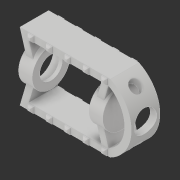
# Autodesk Inventor part: Pedal
Saved by Autodesk Inventor 2019 (Build 230136000, 136)
## iProperties
Created: 2020-06-01
Part Number: Pedal
Material: Generic
Document SubType Name: Modeling
Designer: 18186
Density: 1 g/cm^3
Appearance: Default
Author: 18186
Autodesk Inventor part; units mm, degrees
sketch "Sketch1" plane through (0, 0, 0) normal (0, 0, 1) x (1, 0, 0)
  line L0 (40, -30) -> (-40, -30)
  line L1 (-40, -30) -> (-40, 30) construction
  line L2 (-40, 30) -> (40, 30)
  line L3 (40, 30) -> (40, -30) construction
  line L4 (40, -30) -> (-40, 30) construction
  line L5 (-40, -30) -> (40, 30) construction
  line L6 (40, 30) -> (31.2306, 0)
  line L7 (31.2306, 0) -> (40, -30)
  line L8 (0, 0) -> (0, 5.5495) construction
  line L9 (-40, 30) -> (-31.2306, 0)
  line L10 (-31.2306, 0) -> (-40, -30)
  line L11 (-32.2696, 24.2022) -> (32.2696, 24.2022)
  line L12 (32.2696, 24.2022) -> (25.195, 0)
  line L13 (21.0953, 0) -> (28.6046, 0) construction
  line L14 (-32.2696, -24.2022) -> (32.2696, -24.2022)
  line L15 (32.2696, -24.2022) -> (25.195, 0)
  line L16 (-32.2696, 24.2022) -> (-25.195, 0)
  line L17 (-32.2696, -24.2022) -> (-25.195, 0)
  dimension "d0" = 80
  dimension "d1" = 60
  constraints: 36 end point, 4 symmetric about line, 3 horizontal, 3 parallel, 3 point on line, 2 midpoint, 1 perpendicular, 1 vertical
  measures "d0" distance of L1.end L2.end
  measures "d1" distance of L0.end L1.end
extrude "Extrusion1" add sketch "Sketch1" along normal blind 25.4
ref_plane "Work Plane2" through (-31.2306, 0, 0) normal (-1, 0, 0) x (0, 0, 1)
ref_plane "Work Plane1" through (-31.2306, 0, 0) normal (0, 1, 0) x (0, 0, 1)
sketch "Sketch2" plane through (-31.2306, 0, 0) normal (-1, 0, 0) x (0, 0, 1)
  line L0 (0, 0) -> (25.4, 0) projected
  circle A0 centre (12.7, 0) radius 16.7045
  dimension "d5" = 33.409
  constraints: 1 centre point, 1 midpoint
  measures "d5" diameter of A0
extrude "Extrusion2" add sketch "Sketch2" along normal mid plane 12.0904
sketch "Sketch3" plane through (-37.2758, 0, 12.7) normal (-1, 0, 0) x (0, 0, 1)
  point P0 (-12.7, 0)
sketch "Sketch4" plane through (-37.2758, 0, 12.7) normal (-1, 0, 0) x (0, 0, 1)
  circle A0 centre (0, 0) radius 14.1645
  dimension "d8" = 28.329
  constraints: 1 centre point
  measures "d8" diameter of A0
extrude "Extrusion3" cut sketch "Sketch4" against normal blind 9
sketch "Sketch5" plane through (-40, -30, 0) normal (0, -1, 0) x (1, 0, 0)
  line L0 (40, 25.4) -> (40, 0) construction
  constraints: 2 end point, 1 vertical
sketch "Sketch6" plane through (-40, 30, 0) normal (0, 1, 0) x (1, 0, 0)
  line L0 (40, -25.4) -> (40, 0) construction
  constraints: 2 end point, 1 vertical
ref_plane "Work Plane3" through (0, -30, 25.4) normal (1, 0, 0) x (0, 0, -1)
mirror "Mirror1" about plane through (0, -30, 25.4) normal (1, 0, 0) of "Extrusion2"
sketch "Sketch7" plane through (25.1854, 0, 12.7) normal (-1, 0, 0) x (0, 0, 1)
  circle A0 centre (0, 0) radius 14.1645
  point P0 (-12.7, 0)
  dimension "d11" = 28.329
  constraints: 1 centre point
  measures "d11" diameter of A0
extrude "Extrusion4" cut sketch "Sketch7" against normal blind 9
sketch "Sketch8" plane through (-28.2758, 0, 12.7) normal (-1, 0, 0) x (0, 0, 1)
  circle A0 centre (0, 0) radius 10
  point P0 (-12.7, 0)
  dimension "d14" = 20
  constraints: 1 centre point
  measures "d14" diameter of A0
extrude "Extrusion5" cut sketch "Sketch8" against normal blind 9
sketch "Sketch9" plane through (0, 0, 25.4) normal (0, 0, 1) x (1, 0, 0)
  arc A0 (40, -30) -> (40, 30) centre (25.1772, 0) ccw
  line L0 (32.2696, -24.2022) -> (38.3052, -24.2022) construction
  line L1 (32.2696, 24.2022) -> (38.3052, 24.2022) construction
  arc A1 (38.3052, -24.2022) -> (38.3052, 24.2022) centre (25.1772, 0) ccw
  line L2 (38.3052, -24.2022) -> (40, -30)
  line L3 (38.3052, 24.2022) -> (40, 30)
  point P0 (0, 0)
  constraints: 8 end point, 4 point on circle, 2 centre point, 2 horizontal, 1 concentric
extrude "Extrusion6" add sketch "Sketch9" against normal blind 25.4
ref_plane "Work Plane4" through (62.6758, 0, 12.7) normal (1, 0, 0) x (0, 0, -1)
sketch "Sketch10" plane through (62.6758, 0, 12.7) normal (1, 0, 0) x (0, 0, -1)
  circle A0 centre (0, 0) radius 10
  point P0 (12.7, 0)
  constraints: 1 centre point
extrude "Extrusion7" cut sketch "Sketch10" against normal blind 22.225
ref_plane "Work Plane5" through (40, 30, 0) normal (0.443, 0.8965, 0) x (-0.8965, 0.443, 0)
sketch "Sketch11" plane through (40, 30, 0) normal (0.443, 0.8965, 0) x (-0.8965, 0.443, 0)
  circle A0 centre (-11.6035, 12.5893) radius 5.1558
  point P0 (22.5723, 0)
  constraints: 1 centre point
extrude "Extrusion8" cut sketch "Sketch11" against normal blind 14.2875
ref_plane "Work Plane6" through (-40, 0, 25.4) normal (0, 1, 0) x (1, 0, 0)
mirror "Mirror2" about plane through (-40, 0, 25.4) normal (0, 1, 0) of "Extrusion8"
sketch "Sketch12" plane through (0, 0, 25.4) normal (0, 0, 1) x (1, 0, 0)
  line L0 (-32.2696, -24.2022) -> (-32.2696, -30) construction
  line L1 (-39.1526, -27.1011) -> (44.8049, -27.1011) construction
  line L2 (37.8474, -24.5611) -> (32.7674, -24.5611)
  line L3 (32.7674, -24.5611) -> (32.7674, -29.6411)
  line L4 (32.7674, -29.6411) -> (37.8474, -29.6411)
  line L5 (37.8474, -29.6411) -> (37.8474, -24.5611)
  line L6 (37.8474, -24.5611) -> (32.7674, -29.6411) construction
  line L7 (32.7674, -24.5611) -> (37.8474, -29.6411) construction
  line L8 (32.7674, -27.1011) -> (19.0514, -27.1011) construction
  line L9 (16.5114, -24.5611) -> (21.5914, -24.5611)
  line L10 (21.5914, -24.5611) -> (21.5914, -29.6411)
  line L11 (21.5914, -29.6411) -> (16.5114, -29.6411)
  line L12 (16.5114, -29.6411) -> (16.5114, -24.5611)
  line L13 (16.5114, -24.5611) -> (21.5914, -29.6411) construction
  line L14 (21.5914, -24.5611) -> (16.5114, -29.6411) construction
  line L15 (16.5114, -27.1011) -> (2.7954, -27.1011) construction
  line L16 (0.2554, -24.5611) -> (5.3354, -24.5611)
  line L17 (5.3354, -24.5611) -> (5.3354, -29.6411)
  line L18 (5.3354, -29.6411) -> (0.2554, -29.6411)
  line L19 (0.2554, -29.6411) -> (0.2554, -24.5611)
  line L20 (0.2554, -24.5611) -> (5.3354, -29.6411) construction
  line L21 (5.3354, -24.5611) -> (0.2554, -29.6411) construction
  line L22 (0.2554, -27.1011) -> (-13.4606, -27.1011) construction
  line L23 (-16.0006, -24.5611) -> (-10.9206, -24.5611)
  line L24 (-10.9206, -24.5611) -> (-10.9206, -29.6411)
  line L25 (-10.9206, -29.6411) -> (-16.0006, -29.6411)
  line L26 (-16.0006, -29.6411) -> (-16.0006, -24.5611)
  line L27 (-16.0006, -24.5611) -> (-10.9206, -29.6411) construction
  line L28 (-10.9206, -24.5611) -> (-16.0006, -29.6411) construction
  line L29 (-16.0006, -27.1011) -> (-29.7166, -27.1011) construction
  line L30 (-32.2566, -24.5611) -> (-27.1766, -24.5611)
  line L31 (-27.1766, -24.5611) -> (-27.1766, -29.6411)
  line L32 (-27.1766, -29.6411) -> (-32.2566, -29.6411)
  line L33 (-32.2566, -29.6411) -> (-32.2566, -24.5611)
  line L34 (-32.2566, -24.5611) -> (-27.1766, -29.6411) construction
  line L35 (-27.1766, -24.5611) -> (-32.2566, -29.6411) construction
  point P0 (0, 0)
  point P1 (35.3074, -27.1011)
  dimension "d24" = 5.08
  dimension "d25" = 5.08
  dimension "d26" = 13.716
  dimension "d27" = 5.08
  dimension "d28" = 5.08
  dimension "d29" = 13.716
  dimension "d30" = 5.08
  dimension "d31" = 5.08
  dimension "d32" = 13.716
  dimension "d33" = 5.08
  dimension "d34" = 5.08
  dimension "d35" = 13.716
  dimension "d36" = 5.08
  dimension "d37" = 5.08
  constraints: 72 end point, 14 midpoint, 10 parallel, 7 horizontal, 5 perpendicular, 5 point on line, 2 vertical
  measures "d24" distance of L4.end L3.end
  measures "d25" distance of L3.end L2.end
  measures "d26" distance of L8.start L8.end
  measures "d27" distance of L10.end L11.end
  measures "d28" distance of L9.end L10.end
  measures "d29" distance of L15.start L15.end
  measures "d30" distance of L17.end L18.end
  measures "d31" distance of L16.end L17.end
  measures "d32" distance of L22.start L22.end
  measures "d33" distance of L24.end L25.end
  measures "d34" distance of L23.end L24.end
  measures "d35" distance of L29.start L29.end
  measures "d36" distance of L31.end L32.end
  measures "d37" distance of L30.end L31.end
extrude "Extrusion9" add sketch "Sketch12" along normal blind 2.54
chamfer "Chamfer1" distance 1.5875 angle 45 20 edges at (32.7674, -27.1011, 27.94) (35.3074, -29.6411, 27.94) (37.8474, -27.1011, 27.94) (35.3074, -24.5611, 27.94) (19.0514, -24.5611, 27.94) (16.5114, -27.1011, 27.94) (19.0514, -29.6411, 27.94) (21.5914, -27.1011, 27.94) (2.7954, -24.5611, 27.94) (0.2554, -27.1011, 27.94) (2.7954, -29.6411, 27.94) (5.3354, -27.1011, 27.94) (-13.4606, -24.5611, 27.94) (-10.9206, -27.1011, 27.94) (-13.4606, -29.6411, 27.94) (-16.0006, -27.1011, 27.94) (-29.7166, -24.5611, 27.94) (-27.1766, -27.1011, 27.94) (-29.7166, -29.6411, 27.94) (-32.2566, -27.1011, 27.94)
ref_plane "Work Plane7" through (0, 0, 12.7) normal (0, 0, 1) x (1, 0, 0)
mirror "Mirror3" about plane through (-40, 0, 25.4) normal (0, 1, 0) of "Extrusion9"
mirror "Mirror4" about plane through (0, 0, 12.7) normal (0, 0, 1) of "Extrusion9", "Mirror3"
chamfer "Chamfer2" distance 1.5875 angle 45 40 edges at (32.7674, 27.1011, 27.94) (35.3074, 24.5611, 27.94) (37.8474, 27.1011, 27.94) (35.3074, 29.6411, 27.94) (19.0514, 29.6411, 27.94) (21.5914, 27.1011, 27.94) (19.0514, 24.5611, 27.94) (16.5114, 27.1011, 27.94) (2.7954, 29.6411, 27.94) (0.2554, 27.1011, 27.94) (2.7954, 24.5611, 27.94) (5.3354, 27.1011, 27.94) (-13.4606, 29.6411, 27.94) (-16.0006, 27.1011, 27.94) (-13.4606, 24.5611, 27.94) (-10.9206, 27.1011, 27.94) (-29.7166, 29.6411, 27.94) (-32.2566, 27.1011, 27.94) (-29.7166, 24.5611, 27.94) (-27.1766, 27.1011, 27.94) (-32.2566, 27.1011, -2.54) (-29.7166, 24.5611, -2.54) (-27.1766, 27.1011, -2.54) (-29.7166, 29.6411, -2.54) (-16.0006, 27.1011, -2.54) (-13.4606, 24.5611, -2.54) (-10.9206, 27.1011, -2.54) (-13.4606, 29.6411, -2.54) (0.2554, 27.1011, -2.54) (2.7954, 29.6411, -2.54) (5.3354, 27.1011, -2.54) (2.7954, 24.5611, -2.54) (16.5114, 27.1011, -2.54) (19.0514, 24.5611, -2.54) (21.5914, 27.1011, -2.54) (19.0514, 29.6411, -2.54) (35.3074, 29.6411, -2.54) (37.8474, 27.1011, -2.54) (35.3074, 24.5611, -2.54) (32.7674, 27.1011, -2.54)
chamfer "Chamfer3" distance 1.5875 angle 45 20 edges at (32.7674, -27.1011, -2.54) (35.3074, -24.5611, -2.54) (37.8474, -27.1011, -2.54) (35.3074, -29.6411, -2.54) (16.5114, -27.1011, -2.54) (19.0514, -24.5611, -2.54) (21.5914, -27.1011, -2.54) (19.0514, -29.6411, -2.54) (2.7954, -24.5611, -2.54) (5.3354, -27.1011, -2.54) (2.7954, -29.6411, -2.54) (0.2554, -27.1011, -2.54) (-16.0006, -27.1011, -2.54) (-13.4606, -29.6411, -2.54) (-13.4606, -24.5611, -2.54) (-10.9206, -27.1011, -2.54) (-29.7166, -29.6411, -2.54) (-29.7166, -24.5611, -2.54) (-32.2566, -27.1011, -2.54) (-27.1766, -27.1011, -2.54)
body "Solid1"
